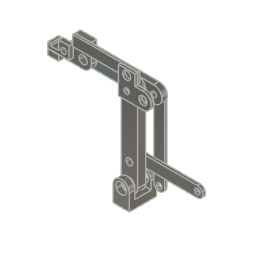
ROBOTARM v1 (Autodesk Fusion 360 design; units mm, degrees)
Autodesk Fusion 360 part; units mm, degrees
sketch "Sketch1" plane through (0, 0, 0) normal (0, 1, 0) x (1, 0, 0)
  line L0 (39.5727, -7.238) -> (62.0727, -7.238)
  line L1 (62.0727, -7.238) -> (62.0727, 4.562)
  line L2 (62.0727, 4.562) -> (39.5727, 4.562)
  line L3 (39.5727, 4.562) -> (39.5727, -7.238)
  dimension "d1" = 22.5
  dimension "d2" = 11.8
  constraint horizontal L0
  constraint vertical L1
  constraint horizontal L2
  constraint vertical L3
  measures "d1" distance of L0.start L0.end
  measures "d2" distance of L0.start L2.end
sketch "Sketch2" plane through (0, 0, 0) normal (0, 1, 0) x (1, 0, 0)
sketch "Sketch3" plane through (0, 0, 0) normal (0, 1, 0) x (1, 0, 0)
  line L0 (6, -3) -> (9, -3)
  line L1 (9, -3) -> (9, 0)
  line L2 (9, 0) -> (6, 0)
  line L3 (6, 0) -> (6, -3)
  circle A0 centre (7.5, -3) radius 1.5
  constraint horizontal L0
  constraint vertical L1
  constraint horizontal L2
  constraint vertical L3
  constraint midpoint L0 A0.centre
  constraint coincident L0.start A0
extrude "Extrude2" add sketch "Sketch3" along normal blind 5 makes body 1
hole "Hole1" at (7.4954, 5, 3.0216) direction (0, -1, 0) diameter 2 depth 5.7 tip angle 118 bodies 1
sketch "Sketch4" plane through (9, 0, 0) normal (1, 0, 0) x (0, 1, 0)
  line L0 (0, 3) -> (0, 0)
  line L1 (0, 0) -> (5, 0)
  line L2 (5, 0) -> (5, 3)
  line L3 (5, 3) -> (0, 3)
  line L4 (1, 4.5) -> (4, 4.5)
  line L5 (4, 4.5) -> (4, 1.5)
  line L6 (4, 1.5) -> (1, 1.5)
  line L7 (1, 1.5) -> (1, 4.5)
  constraint horizontal L4
  constraint vertical L5
  constraint horizontal L6
  constraint vertical L7
extrude "Extrude3" cut sketch "Sketch4" against normal blind 3.4 contours L3 L4 L5 L7 | L3 L5 L6 L7 bodies 1
sketch "Sketch5" plane through (0, 0, 0) normal (0, 1, 0) x (1, 0, 0)
  line L0 (6, -3) -> (9, -3)
  line L1 (9, -3) -> (9, -18)
  line L2 (9, -18) -> (6, -18)
  line L3 (6, -18) -> (6, -3)
  circle A0 centre (7.5, -3) radius 1.5
  constraint horizontal L0
  constraint vertical L1
  constraint horizontal L2
  constraint vertical L3
  constraint midpoint L0 A0.centre
move_body "Move4" bodies 1 to x (1, 0, 0) y (0, 1, 0) z (0, 0, 1) at (0, -3, 0)
extrude "Extrude4" add sketch "Sketch5" against normal blind 1.5 separate body makes body 2
extrude "Extrude5" add 1 faces at (8, 0, 13) along direction (0, 1, 0) blind 0.5 on bodies 2 bodies 1 2
sketch "Sketch6" plane through (0, 0, 0) normal (0, 1, 0) x (1, 0, 0)
  circle A0 centre (7.5, -18) radius 1.5
extrude "Extrude6" add sketch "Sketch6" along normal blind 0.5 bodies 1
extrude "Extrude7" add 1 faces at (7.4626, 0, 18.4986) along direction (0, -1, 0) blind 1.5 on bodies 1 bodies 1
extrude "Extrude8" cut 3 faces at (7.4626, 0.5, 18.4986) (7.4626, 0.5, 7.5014) (7.4626, 0.5, 17.3524) along direction (0, -1, 0) blind 0.5 on bodies 1 bodies 1
sketch "Sketch7" plane through (0, 0, 0) normal (0, 1, 0) x (1, 0, 0)
  circle A0 centre (7.5, -18) radius 1.5
  line L0 (7.5, -19.5) -> (-1.5, -19.5)
  line L1 (-1.5, -19.5) -> (-1.5, -16.5)
  line L2 (-1.5, -16.5) -> (7.5, -16.5)
  line L3 (7.5, -16.5) -> (7.5, -19.5)
  circle A1 centre (-1.5, -18) radius 1.5
  constraint horizontal L0
  constraint vertical L1
  constraint horizontal L2
  constraint vertical L3
  constraint coincident A0 L0.start
  constraint midpoint L1 A1.centre
extrude "Extrude9" add sketch "Sketch7" along normal blind 1 separate body makes body 3
sketch "Sketch8" plane through (0, 0, 0) normal (0, 1, 0) x (1, 0, 0)
  line L0 (7.5, -16.5) -> (10.4989, -16.5)
  line L1 (10.4989, -16.5) -> (10.4989, -19.5)
  line L2 (10.4989, -19.5) -> (7.5, -19.5)
  line L3 (7.5, -19.5) -> (7.5, -16.5)
  circle A0 centre (10.4989, -18) radius 1.5011
  constraint horizontal L0
  constraint vertical L1
  constraint horizontal L2
  constraint vertical L3
  constraint midpoint L1 A0.centre
extrude "Extrude10" add sketch "Sketch8" along normal blind 1 bodies 1 3
sketch "Sketch9" plane through (0, 0, 0) normal (0, 1, 0) x (1, 0, 0)
  circle A0 centre (7.5, -6.5) radius 1
  line L0 (7.5, -7.5) -> (18.5, -7.5)
  line L1 (18.5, -7.5) -> (18.5, -5.5)
  line L2 (18.5, -5.5) -> (7.5, -5.5)
  line L3 (7.5, -5.5) -> (7.5, -7.5)
  circle A1 centre (18.5, -6.5) radius 1
  constraint horizontal L0
  constraint vertical L1
  constraint horizontal L2
  constraint vertical L3
  constraint coincident A0 L0.start
extrude "Extrude11" add sketch "Sketch9" along normal blind 0.5 separate body makes body 4
sketch "Sketch10" plane through (0, 0, 0) normal (0, 1, 0) x (1, 0, 0)
sketch "Sketch11" plane through (0, 0, 0) normal (0, 1, 0) x (1, 0, 0)
sketch "Sketch12" plane through (0, 0, 0) normal (0, 1, 0) x (1, 0, 0)
  line L0 (7.5, -19) -> (5.5, -19)
  line L1 (5.5, -19) -> (5.5, -17)
  line L2 (5.5, -17) -> (7.5, -17)
  line L3 (7.5, -17) -> (7.5, -19)
  circle A0 centre (5.5, -18) radius 1
  circle A1 centre (-1.5, -18) radius 1
  line L4 (-1.5, -19) -> (-3.5, -19)
  line L5 (-3.5, -19) -> (-3.5, -17)
  line L6 (-3.5, -17) -> (-1.5, -17)
  line L7 (-1.5, -17) -> (-1.5, -19)
  line L8 (-2.5, -18) -> (-0.5, -18)
  line L9 (-0.5, -18) -> (-0.5, -20)
  line L10 (-0.5, -20) -> (-2.5, -20)
  line L11 (-2.5, -20) -> (-2.5, -18)
  constraint horizontal L0
  constraint vertical L1
  constraint horizontal L2
  constraint vertical L3
  constraint midpoint L1 A0.centre
  constraint coincident L1.end A0
  constraint horizontal L4
  constraint vertical L5
  constraint horizontal L6
  constraint vertical L7
  constraint coincident A1 L4.start
  constraint horizontal L8
  constraint vertical L9
  constraint horizontal L10
  constraint vertical L11
  constraint coincident A1 L8.start
sketch "Sketch13" plane through (0, 0, 0) normal (0, 1, 0) x (1, 0, 0)
  circle A0 centre (-1.5, -20) radius 1
sketch "Sketch14" plane through (0, 0, 0) normal (0, 1, 0) x (1, 0, 0)
sketch "Sketch15" plane through (0, 0, 0) normal (0, 1, 0) x (1, 0, 0)
  line L0 (-3.5, -17) -> (-5, -17)
  line L1 (-5, -17) -> (-5, -18)
  line L2 (-5, -18) -> (-3.5, -18)
  line L3 (-3.5, -18) -> (-3.5, -17)
  line L4 (-5, -17) -> (-6, -17)
  line L5 (-6, -17) -> (-6, -17.25)
  line L6 (-4.25, -19) -> (-5, -19)
  line L7 (-5, -19) -> (-5, -17)
  arc A0 (-6, -17.25) -> (-4.25, -19) centre (-4.25, -17.25) ccw
  dimension "d37" = 1.75
  constraint horizontal L0
  constraint vertical L1
  constraint horizontal L2
  constraint vertical L3
  constraint horizontal L4
  constraint vertical L5
  constraint horizontal L6
  constraint vertical L7
  constraint tangent L5 A0
  constraint tangent L6 A0
  measures "d37" radius of A0
sketch "Sketch16" plane through (0, 0, 0) normal (0, 1, 0) x (1, 0, 0)
  circle A0 through (8.1, -6.5, 0.7) (7.2, -5.9804, 0.7) (7.2, -7.0196, 0.7)
extrude "Extrude13" cut sketch "Sketch16" against normal blind 3.5 contours A0 in plane through (0, 0.7, 0) normal (0, 1, 0) bodies 1 4
sketch "Sketch17" plane through (0, 0, 0) normal (0, 1, 0) x (1, 0, 0)
  circle A0 through (11.5, -18, 1) (10, -17.134, 1) (10, -18.866, 1)
sketch "Sketch18" plane through (0, 0, 0) normal (0, 1, 0) x (1, 0, 0)
  line L0 (11.5, -17.9965, 1) -> (9.5, -17.9965, 1)
  line L1 (9.5, -17.9965, 1) -> (9.5, -3, 1)
  line L2 (9.5, -3, 1) -> (11.5, -3, 1)
  line L3 (11.5, -3, 1) -> (11.5, -17.9965, 1)
  circle A0 through (11.5, -3, 1) (10, -2.134, 1) (10, -3.866, 1)
sketch "Sketch19" plane through (0, 0, 0) normal (0, 1, 0) x (1, 0, 0)
sketch "Sketch20" plane through (0, -1.5, 0) normal (0, -1, 0) x (1, 0, 0)
  arc A0 (-0.5, 20) -> (-2.5, 20) centre (-1.5, 20) ccw
  line L0 (-2.5, 20) -> (-2.5, 19)
  line L1 (-2.5, 19) -> (-3.5, 19)
  line L2 (-3.5, 19) -> (-3.5, 18)
  line L3 (-3.5, 18) -> (-5, 18)
  line L4 (-5, 18) -> (-5, 18.8311)
  arc A1 (-5, 18.8311) -> (-6, 17.25) centre (-4.25, 17.25) ccw
  line L5 (-6, 17.25) -> (-6, 17)
  line L6 (-6, 17) -> (-1.5, 17)
  arc A2 (-1.5, 17) -> (-0.5, 18) centre (-1.5, 18) ccw
  line L7 (-0.5, 18) -> (-0.5, 20)
  circle A3 centre (-1.5, 18) radius 0.7
  constraint concentric A2 A3
extrude "Extrude15" add sketch "Sketch17" sketch "Sketch18" along normal blind 0.4 separate body contours A0 in plane through (0, 1, 0) normal (0, 1, 0) of sketch 2 contours L0 L1 L3 A0 | L2 A0 | L2 A0 in plane through (0, 1, 0) normal (0, 1, 0) makes body 5
sketch "Sketch21" plane through (0, -1, 0) normal (0, -1, 0) x (1, 0, 0)
sketch "Sketch22" plane through (0, -1.5, 0) normal (0, -1, 0) x (1, 0, 0)
  circle A0 centre (7.5, 6.5) radius 0.6
  line L0 (9, 3) -> (9, 18)
  arc A1 (9, 18) -> (6, 18) centre (7.5, 18) ccw
  line L1 (6, 18) -> (6, 3)
  arc A2 (6, 3) -> (7.5, 1.5) centre (7.5, 3) ccw
  arc A3 (7.5, 1.5) -> (9, 3) centre (7.5, 3) ccw
  circle A4 centre (7.5, 18) radius 0.5
  constraint concentric A1 A4
extrude "Extrude17" cut sketch "Sketch22" against normal blind 5.1 contours A4 bodies 1
sketch "Sketch23" plane through (0, 0, 0) normal (0, -1, 0) x (1, 0, 0)
  arc A0 (7.5, 19.5) -> (6, 18) centre (7.5, 18) ccw
  line L0 (7.5, 19.5) -> (-1.5, 19.5)
  arc A1 (-1.5, 19.5) -> (-1.5, 16.5) centre (-1.5, 18) ccw
  line L1 (-1.5, 16.5) -> (6, 16.5)
  line L2 (6, 16.5) -> (6, 18)
  circle A2 centre (-1.5, 18) radius 1.5
  line L3 (-1.5, 19.5) -> (-5, 19.5)
  line L4 (-5, 19.5) -> (-5, 16.5)
  line L5 (-5, 16.5) -> (-1.5, 16.5)
  line L6 (-1.5, 16.5) -> (-1.5, 19.5)
  line L7 (-3, 18) -> (0, 18)
  line L8 (0, 18) -> (0, 21.5)
  line L9 (0, 21.5) -> (-3, 21.5)
  line L10 (-3, 21.5) -> (-3, 18)
  circle A3 centre (-1.5, 20.5) radius 0.8
  circle A4 centre (-1.5, 18) radius 0.75
  constraint concentric A1 A2
  constraint coincident L0.end A2
  constraint horizontal L3
  constraint vertical L4
  constraint horizontal L5
  constraint vertical L6
  constraint coincident L0.end A1.start
  constraint horizontal L7
  constraint vertical L8
  constraint horizontal L9
  constraint vertical L10
  constraint midpoint A1 L7.start
  constraint concentric A1 A4
extrude "Extrude18" add sketch "Sketch23" along normal blind 1 separate body contours L0 A2 L8 | L0 L3 L8 L9 L10 | A1 A2 L6 L7 A4 | A1 A2 L3 L10 | A2 L6 L7 A4 | A2 L6 L7 A4 | A1 A2 L3 L4 L5 L10 | A1 A2 L6 L7 A4 makes body 6
sketch "Sketch24" plane through (0, 0, 0) normal (0, -1, 0) x (1, 0, 0)
  arc A0 (7.5, 19.5) -> (6, 18) centre (7.5, 18) ccw
  line L0 (7.5, 19.5) -> (-1.5, 19.5)
  arc A1 (-1.5, 19.5) -> (-1.5, 16.5) centre (-1.5, 18) ccw
  line L1 (-1.5, 16.5) -> (6, 16.5)
  line L2 (6, 16.5) -> (6, 18)
sketch "Sketch25" plane through (0, -1.5, 0) normal (0, -1, 0) x (1, 0, 0)
  circle A0 centre (7.5, 18) radius 0.5
  circle A1 centre (7.5, 6.5) radius 0.6
  line L0 (9, 3) -> (9, 18)
  arc A2 (9, 18) -> (6, 18) centre (7.5, 18) ccw
  line L1 (6, 18) -> (6, 3)
  arc A3 (6, 3) -> (7.5, 1.5) centre (7.5, 3) ccw
  arc A4 (7.5, 1.5) -> (9, 3) centre (7.5, 3) ccw
  line L2 (6, 16.5) -> (10.5, 16.5)
  line L3 (10.5, 19.5) -> (6, 19.5)
  line L4 (6, 19.5) -> (6, 16.5)
  arc A5 (12, 18) -> (10.5, 19.5) centre (10.5, 18) ccw
  arc A6 (10.5, 16.5) -> (12, 18) centre (10.5, 18) ccw
  line L5 (6, 19.5) -> (9, 19.5)
  line L6 (9, 19.5) -> (9, 21.5)
  line L7 (9, 21.5) -> (6, 21.5)
  line L8 (6, 21.5) -> (6, 19.5)
  circle A7 centre (7.5, 20.5) radius 0.75
  circle A8 centre (10.5, 18) radius 0.75
  dimension "d52" = 1.5
  constraint horizontal L2
  constraint horizontal L3
  constraint vertical L4
  constraint coincident L1 L2.start
  constraint tangent L3 A5
  constraint tangent L2 A6
  constraint equal A5 A6
  constraint coincident A5.start A6.end
  constraint horizontal L5
  constraint vertical L6
  constraint horizontal L7
  constraint vertical L8
  constraint concentric A5 A8
  measures "d52" radius of A5
sketch "Sketch26" plane through (0, -1.5, 0) normal (0, -1, 0) x (1, 0, 0)
extrude "Extrude19" add sketch "Sketch25" along normal blind 0.5 separate body contours L0 A2 L1 L2 L4 | L0 A2 L2 L3 A5 A6 L5 | L3 L5 L6 L7 L8 | A2 L3 L4 L5 makes body 7
sketch "Sketch27" plane through (0, 1, 0) normal (0, 1, 0) x (-1, 0, 0)
  circle A0 centre (-7.5, 18) radius 0.5
  line L0 (-10.4412, 16.5) -> (1.5, 16.5)
  arc A1 (1.5, 16.5) -> (1.5, 19.5) centre (1.5, 18) ccw
  line L1 (1.5, 19.5) -> (-10.4412, 19.5)
  arc A2 (-10.4412, 19.5) -> (-10.4412, 16.5) centre (-10.4989, 18) ccw
  line L2 (-9, 21.5, -2.05) -> (3, 21.5, -2.05)
  line L3 (3, 21.5, -2.05) -> (3, 19.6, -2.05)
  line L4 (3, 19.6, -2.05) -> (-9, 19.6, -2.05)
  line L5 (-9, 19.6, -2.05) -> (-9, 21.5, -2.05)
extrude "Extrude20" add sketch "Sketch27" against normal blind 0.4 separate body contours L2 L3 L4 L5 in plane through (0, -1.05, 0) normal (0, 1, 0) makes body 8
sketch "Sketch28" plane through (-5, 0, 0) normal (-1, 0, 0) x (0, -1, 0)
  line L0 (0, 19.5) -> (0, 16.5)
  line L1 (0, 16.5) -> (1, 16.5)
  line L2 (1, 16.5) -> (1, 19.5)
  line L3 (1, 19.5) -> (0, 19.5)
  line L4 (0, 16.5) -> (2, 16.5)
  line L5 (2, 16.5) -> (2, 17.5)
  line L6 (2, 17.5) -> (0, 17.5)
  line L7 (0, 17.5) -> (0, 16.5)
  constraint horizontal L4
  constraint vertical L5
  constraint horizontal L6
  constraint vertical L7
  constraint coincident L0.end L1.start
extrude "Extrude21" add sketch "Sketch28" along normal blind 2 contours L0 L1 L2 L4 L6 L7 | L2 L4 L5 L6 bodies 6
fillet "Fillet1" radius 1.5 1 edges at (-5, -0.5, 19.5) on bodies 6
sketch "Sketch29" plane through (0, -1, 0) normal (0, -1, 0) x (1, 0, 0)
  arc A0 (-3.5, 19.5) -> (-5, 18) centre (-3.5, 18) ccw
  line L0 (-5, 18) -> (-5, 17.5)
  line L1 (-5, 17.5) -> (-5, 16.5)
  line L2 (-5, 16.5) -> (-1.5, 16.5)
  arc A1 (-1.5, 16.5) -> (0, 18) centre (-1.5, 18) ccw
  line L3 (0, 18) -> (0, 21.5)
  line L4 (0, 21.5) -> (-3, 21.5)
  line L5 (-3, 21.5) -> (-3, 19.5)
  line L6 (-3, 19.5) -> (-3.5, 19.5)
  circle A2 centre (-1.5, 20.5) radius 0.8
  circle A3 centre (-1.5, 18) radius 0.75
  line L7 (-7, 18.5) -> (-6.5, 18.5)
  line L8 (-6.5, 18.5) -> (-6.5, 17.5)
  line L9 (-6.5, 17.5) -> (-7, 17.5)
  line L10 (-7, 17.5) -> (-7, 18.5)
  line L11 (-6.5, 18.1) -> (-5, 18.1)
  line L12 (-5, 18.1) -> (-5, 17.5)
  line L13 (-5, 17.5) -> (-6.5, 17.5)
  line L14 (-6.5, 17.5) -> (-6.5, 18.1)
  line L15 (-5, 17.5) -> (-3.1, 17.5)
  line L16 (-3.1, 17.5) -> (-3.1, 19.8)
  line L17 (-3.1, 19.8) -> (-5, 19.8)
  line L18 (-5, 19.8) -> (-5, 17.5)
  constraint horizontal L7
  constraint vertical L8
  constraint horizontal L9
  constraint vertical L10
  constraint horizontal L11
  constraint vertical L12
  constraint horizontal L13
  constraint vertical L14
  constraint coincident L0.end L1.start
  constraint coincident L8 L11.start
  constraint horizontal L15
  constraint vertical L16
  constraint horizontal L17
  constraint vertical L18
move_body "Move5" bodies 5 6 8 7 1 4 to x (1, 0, 0) y (0, 1, 0) z (0, 0, 1) at (0, 0.2, -0.1)
extrude "Extrude22" add sketch "Sketch29" along normal blind 0.8 separate body contours A0 L0 L6 L12 L15 L16 L18 | A0 L6 L12 L16 L17 L18 | L0 L8 L11 L12 L13 L14 L18 | L7 L8 L9 L10 L14 makes body 9
sketch "Sketch30" plane through (0, -1, 0) normal (0, 1, 0) x (-1, 0, 0)
  line L0 (3.1, 17.5) -> (7, 17.5)
  line L1 (7, 17.5) -> (7, 18.5)
  line L2 (7, 18.5) -> (6.5, 18.5)
  line L3 (6.5, 18.5) -> (6.5, 18.1)
  line L4 (6.5, 18.1) -> (5, 18.1)
  line L5 (5, 18.1) -> (5, 19.8)
  line L6 (5, 19.8) -> (3.1, 19.8)
  line L7 (3.1, 19.8) -> (3.1, 17.5)
  line L8 (5.0272, 18.1) -> (7, 18.1)
  line L9 (7, 18.1) -> (7, 17.5)
  line L10 (7, 17.5) -> (5.0272, 17.5)
  line L11 (5.0272, 17.5) -> (5.0272, 18.1)
  line L12 (6.5, 18.1) -> (7, 18.1)
  line L13 (7, 18.1) -> (7, 18.5)
  line L14 (7, 18.5) -> (6.5, 18.5)
  line L15 (6.5, 18.5) -> (6.5, 18.1)
  constraint horizontal L8
  constraint vertical L9
  constraint horizontal L10
  constraint vertical L11
  constraint coincident L0.end L1.start
  constraint coincident L4 L8.start
  constraint horizontal L12
  constraint vertical L13
  constraint horizontal L14
  constraint vertical L15
  constraint coincident L1.end L2.start
  constraint coincident L3.end L4.start
extrude "Extrude23" add sketch "Sketch30" along normal blind 1.2 contours L0 L1 L4 L8 L9 L10 L11 L12 | L1 L2 L3 L8 L12 L13 L14 L15 bodies 9
sketch "Sketch31" plane through (0, 1.6, 0) normal (0, 1, 0) x (-1, 0, 0)
  arc A0 (-9.5, 17.8965) -> (-11.5, 17.8965) centre (-10.5, 17.9) ccw
  line L0 (-11.5, 17.8965) -> (-11.5, 2.9)
  arc A1 (-11.5, 2.9) -> (-9.5, 2.9) centre (-10.5, 2.9) ccw
  line L1 (-9.5, 2.9) -> (-9.5, 17.8965)
  circle A2 centre (-10.5, 17.9) radius 0.5
  constraint concentric A0 A2
extrude "Extrude24" cut sketch "Sketch31" against normal blind 4.1 contours A2 bodies 1 5
sketch "Sketch32" plane through (0, 1.6, 0) normal (0, 1, 0) x (-1, 0, 0)
  circle A0 centre (-10.5, 17.9) radius 0.5
  arc A1 (-9.5, 17.8965) -> (-11.5, 17.8965) centre (-10.5, 17.9) ccw
  line L0 (-11.5, 17.8965) -> (-11.5, 2.9)
  arc A2 (-11.5, 2.9) -> (-9.5, 2.9) centre (-10.5, 2.9) ccw
  line L1 (-9.5, 2.9) -> (-9.5, 17.8965)
  circle A3 centre (-10.5, 2.8) radius 0.5
extrude "Extrude25" cut sketch "Sketch32" against normal blind 6.9 contours A3 bodies 5
sketch "Sketch33" plane through (0, -0.8, 0) normal (0, -1, 0) x (1, 0, 0)
  arc A0 (-3.5, 19.4) -> (-5, 17.9) centre (-3.5, 17.9) ccw
  line L0 (-5, 17.9) -> (-5, 17.4)
  line L1 (-5, 17.4) -> (-5, 16.4)
  line L2 (-5, 16.4) -> (-1.5, 16.4)
  arc A1 (-1.5, 16.4) -> (0, 17.9) centre (-1.5, 17.9) ccw
  line L3 (0, 17.9) -> (0, 21.4)
  line L4 (0, 21.4) -> (-3, 21.4)
  line L5 (-3, 21.4) -> (-3, 19.4)
  line L6 (-3, 19.4) -> (-3.5, 19.4)
  circle A2 centre (-1.5, 20.4) radius 0.8
  circle A3 centre (-1.5, 17.9) radius 0.75
  circle A4 centre (-1.5, 17.9) radius 0.75
  constraint concentric A1 A4
extrude "Extrude26" cut sketch "Sketch33" against normal blind 3.8 contours A3 A4 bodies 1
sketch "Sketch34" plane through (0, 0, 0) normal (0, 1, 0) x (1, 0, 0)
  circle A0 through (8.5, -2.92, 0.4) (7, -2.054, 0.4) (7, -3.786, 0.4)
extrude "Extrude27" cut sketch "Sketch34" against normal blind 2 contours A0 in plane through (0, 0.4, 0) normal (0, 1, 0) bodies 1
sketch "Sketch35" plane through (0, -1.8, 0) normal (0, -1, 0) x (1, 0, 0)
  line L0 (-7, 17.5) -> (-3.1, 17.5)
  line L1 (-3.1, 17.5) -> (-3.1, 19.8)
  line L2 (-3.1, 19.8) -> (-5, 19.8)
  line L3 (-5, 19.8) -> (-5, 18.1)
  line L4 (-5, 18.1) -> (-6.5, 18.1)
  line L5 (-6.5, 18.1) -> (-6.5, 18.5)
  line L6 (-6.5, 18.5) -> (-7, 18.5)
  line L7 (-7, 18.5) -> (-7, 17.5)
  circle A0 centre (-4.1, 18.5) radius 0.5
extrude "Extrude28" cut sketch "Sketch35" against normal blind 3.5 contours A0 bodies 6 9
sketch "Sketch36" plane through (0, 0.7, 0) normal (0, 1, 0) x (-1, 0, 0)
  circle A0 centre (-7.5, 6.4) radius 0.6
  arc A1 (-18.5, 7.4) -> (-18.5, 5.4) centre (-18.5, 6.4) ccw
  line L0 (-18.5, 5.4) -> (-7.5, 5.4)
  arc A2 (-7.5, 5.4) -> (-7.5, 7.4) centre (-7.5, 6.4) ccw
  line L1 (-7.5, 7.4) -> (-18.5, 7.4)
  circle A3 centre (-18.5, 6.4) radius 0.5
  constraint concentric A1 A3
extrude "Extrude29" cut sketch "Sketch36" against normal blind 2 contours A3 bodies 4
